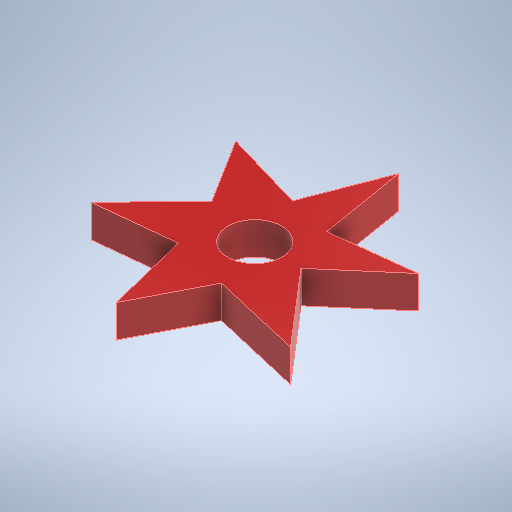
# Autodesk Inventor part: palonnier
Saved by Autodesk Inventor 2026.2 (Build 302298010, 298A)
## iProperties
Created: 2026-04-23
Part Number: palonnier
Material: Générique
Document SubType Name: Modeling
Designer: Genon
Density: 1 g/cm^3
Appearance: Rouge
Author: Genon
Autodesk Inventor part; units mm, degrees
ref_plane "YZ Plane" through (0, 0, 0) normal (1, 0, 0) x (0, 1, 0)
ref_plane "XZ Plane" through (0, 0, 0) normal (0, 1, 0) x (-1, 0, 0)
ref_plane "XY Plane" through (0, 0, 0) normal (0, 0, 1) x (1, 0, 0)
sketch "Esquisse1" plane through (0, 0, 0) normal (1, 0, 0) x (0, 1, 0)
  line L0 (615.5373, -142.1522) -> (811.8285, -142.1522) construction
  line L1 (811.8285, -142.1522) -> (811.8285, -230.5611) construction
  line L2 (811.8285, -230.5611) -> (615.5373, -230.5611) construction
  line L3 (615.5373, -230.5611) -> (615.5373, -142.1522) construction
  circle A0 centre (714.0804, -164.9097) radius 9.3044
  circle A1 centre (714.0804, -164.9097) radius 12.8446
  arc A2 (718.2667, -201.6616) -> (719.1833, -202.8097) centre (719.23, -201.8325) ccw
  arc A3 (719.6606, -209.9141) -> (719.248, -210.7518) centre (719.7361, -210.4718) ccw
  arc A4 (713.6782, -215.3851) -> (712.2032, -215.3703) centre (712.9331, -216.1323) ccw
  line L4 (711.5826, -198.3788) -> (715.3474, -192.8257)
  line L5 (715.3474, -192.8257) -> (719.8038, -195.0511)
  line L6 (719.8038, -195.0511) -> (718.2667, -201.6616)
  line L7 (719.1833, -202.8097) -> (725.8864, -202.9912)
  line L8 (725.8864, -202.9912) -> (726.1597, -208.1294)
  line L9 (726.1597, -208.1294) -> (719.6606, -209.9141)
  line L10 (719.248, -210.7518) -> (722.051, -216.9958)
  line L11 (722.051, -216.9958) -> (717.7376, -219.4332)
  line L12 (717.7376, -219.4332) -> (713.6782, -215.3851)
  line L13 (712.2032, -215.3703) -> (708.5343, -221.0039)
  line L14 (708.5343, -221.0039) -> (704.0426, -218.7609)
  line L15 (704.0426, -218.7609) -> (705.4927, -212.5247)
  line L16 (704.6548, -211.4369) -> (698.081, -211.076)
  line L17 (698.081, -211.076) -> (698.1175, -205.8223)
  line L18 (698.1175, -205.8223) -> (703.9597, -204.218)
  line L19 (704.461, -202.9923) -> (701.4433, -196.9238)
  line L20 (701.4433, -196.9238) -> (705.5988, -194.2119)
  line L21 (705.5988, -194.2119) -> (709.8549, -198.4562)
  arc A5 (719.8038, -195.0511) -> (715.3474, -192.8257) centre (717.4272, -194.2357) ccw
  arc A6 (726.1597, -208.1294) -> (725.8864, -202.9912) centre (725.4624, -205.5902) ccw
  arc A7 (717.7376, -219.4332) -> (722.051, -216.9958) centre (719.7814, -218.0147) ccw
  arc A8 (704.0426, -218.7609) -> (708.5343, -221.0039) centre (706.417, -219.625) ccw
  arc A9 (698.1175, -205.8223) -> (698.081, -211.076) centre (698.2252, -208.45) ccw
  arc A10 (705.5988, -194.2119) -> (701.4433, -196.9238) centre (703.68, -195.8115) ccw
  arc A11 (709.8549, -198.4562) -> (711.5826, -198.3788) centre (710.6833, -197.6255) ccw
  arc A12 (703.9597, -204.218) -> (704.461, -202.9923) centre (703.6717, -203.3848) ccw
  arc A13 (705.4927, -212.5247) -> (704.6548, -211.4369) centre (704.6286, -212.3238) ccw
  point P0 (0, 0)
  constraints: 38 end point, 24 point on circle, 14 centre point, 10 tangent, 4 parallel, 1 coincident, 2 other
extrude "Extrusion1" add sketch "Esquisse1" against normal blind 3 contours A2 L7 L8 L9 A3 L10 L11 L12 A4 L13 L14 L15 A13 L16 L17 L18 A12 L19 L20 L21 A11 L4 L5 L6 | L5 A5 | A6 L8 | L20 A10 | A7 L11 | L17 A9 | A8 L14
sketch "Esquisse17" plane through (-3, 0, 0) normal (-1, 0, 0) x (0, 0, 1)
  circle A0 centre (-207.1899, 711.5984) radius 2.5
  point P0 (0, 0)
  dimension "d66" = 5
  constraints: 1 centre point
  measures "d66" diameter of A0
extrude "Extrusion11" cut sketch "Esquisse17" against normal blind 10
sketch "Esquisse18" plane through (-3, 0, 0) normal (-1, 0, 0) x (0, 0, 1)
  circle A0 centre (-207.1899, 711.5984) radius 2.5 projected
  line L0 (-208.7203, 700.3139) -> (-205.4181, 706.7422)
  line L1 (-205.4181, 706.7422) -> (-197.0964, 704.8049)
  line L2 (-197.0964, 704.8049) -> (-202.9234, 711.5984)
  line L3 (-202.9234, 711.5984) -> (-197.0964, 716.5964)
  line L4 (-197.0964, 716.5964) -> (-204.6899, 715.7243)
  line L5 (-204.6899, 715.7243) -> (-205.9905, 723.6937)
  line L6 (-205.9905, 723.6937) -> (-208.7203, 716.5964)
  line L7 (-208.7203, 716.5964) -> (-216.1173, 718.7623)
  line L8 (-216.1173, 718.7623) -> (-212.4188, 712.8623)
  line L9 (-212.4188, 712.8623) -> (-217.8785, 707.1825)
  line L10 (-217.8785, 707.1825) -> (-210.6003, 707.9486)
  line L11 (-210.6003, 707.9486) -> (-208.7203, 700.3139)
  circle A1 centre (-207.1899, 711.5984) radius 19.7592
  point P0 (0, 0)
  constraints: 24 end point, 1 centre point, 1 coincident, 1 perpendicular, 1 point on line
extrude "Extrusion12" cut sketch "Esquisse18" against normal blind 10 contours A1
